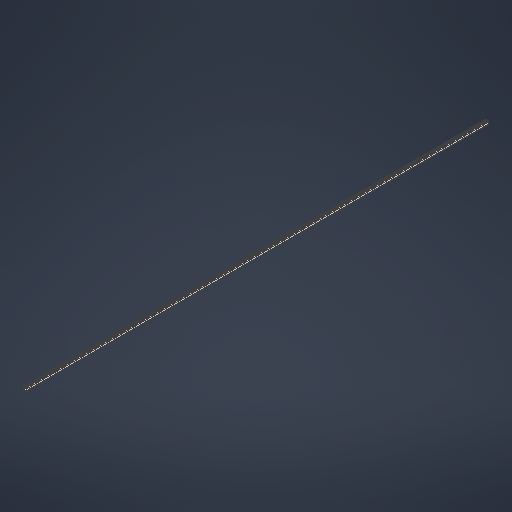
# Autodesk Inventor part: SP40-02 HOJA PUERTA BATIENTE INT - EXT
Saved by Autodesk Inventor 2025 (Build 290162000, 162)
## iProperties
Created: 2026-01-18
Part Number: SP40-02 HOJA PUERTA BATIENTE INT - EXT
Material: Aluminio
Document SubType Name: Modeling
Designer: ROLANDO
Density: 2.7 g/cm^3
Appearance: Satinado
Author: ROLANDO
Autodesk Inventor part; units mm, degrees
ref_plane "YZ Plane" through (0, 0, 0) normal (1, 0, 0) x (0, 1, 0)
ref_plane "XZ Plane" through (0, 0, 0) normal (0, 1, 0) x (-1, 0, 0)
ref_plane "XY Plane" through (0, 0, 0) normal (0, 0, 1) x (1, 0, 0)
sketch "Boceto1" plane through (0, 0, 0) normal (0, 0, 1) x (1, 0, 0)
  line L0 (33.1157, -5.4655) -> (33.1157, 13.4345)
  line L1 (32.6157, 13.9345) -> (-3.8843, 13.9345)
  line L2 (-4.3843, 13.4345) -> (-4.3843, -5.4655)
  line L3 (-3.8843, 15.3345) -> (32.6157, 15.3345)
  line L4 (34.5157, 29.7345) -> (34.5157, -11.2655)
  line L5 (-5.7843, -28.8655) -> (-5.7843, 25.5945)
  line L6 (33.1157, 15.8345) -> (33.1157, 28.3345)
  line L7 (34.5157, 29.7345) -> (20.3157, 29.7345)
  line L8 (20.3157, 29.7345) -> (20.3157, 28.0945)
  line L9 (24.1157, 28.3345) -> (24.1157, 21.8345)
  line L10 (25.5157, 20.4345) -> (25.5157, 28.3345)
  line L11 (25.5157, 20.4345) -> (20.3157, 20.4345)
  line L12 (20.3157, 20.4345) -> (20.3157, 22.0745)
  line L13 (21.7157, 21.8345) -> (24.1157, 21.8345)
  line L14 (21.7157, 23.0845) -> (21.0099, 23.0845)
  line L15 (21.0099, 23.0845) -> (20.3157, 22.0745)
  line L16 (21.7157, 27.0845) -> (21.0099, 27.0845)
  line L17 (-4.3843, 15.8345) -> (-4.3843, 22.8345)
  line L18 (-4.3843, 22.8345) -> (-2.8843, 22.8345)
  line L19 (-2.8843, 22.8345) -> (-2.8843, 25.5945)
  line L20 (-1.6443, 29.7345) -> (6.5157, 29.7345)
  line L21 (5.0777, 28.3345) -> (-0.1443, 28.3345)
  line L22 (6.5157, 29.7345) -> (6.5157, 27.2345)
  line L23 (6.5157, 27.2345) -> (5.8057, 27.2345)
  line L24 (5.8057, 27.2345) -> (5.0777, 28.3345)
  line L25 (33.1157, -7.8655) -> (33.1157, -11.2655)
  line L26 (33.6157, -11.7655) -> (34.0157, -11.7655)
  line L27 (22.5157, -7.3655) -> (22.5157, -10.3655)
  line L28 (23.9157, -11.7655) -> (23.9157, -7.8655)
  line L29 (1.1157, -7.8655) -> (1.1157, -11.7655)
  line L30 (2.5157, -10.3655) -> (2.5157, -7.3655)
  line L31 (2.5157, -10.3655) -> (5.0157, -10.3655)
  line L32 (5.0157, -10.3655) -> (5.0157, -11.7655)
  line L33 (5.0157, -11.7655) -> (1.1157, -11.7655)
  line L34 (22.5157, -10.3655) -> (20.0157, -10.3655)
  line L35 (20.0157, -10.3655) -> (20.0157, -11.7655)
  line L36 (20.0157, -11.7655) -> (23.9157, -11.7655)
  line L37 (21.4157, -5.4655) -> (21.4157, -4.5655)
  line L38 (21.4157, -4.5655) -> (3.6157, -4.5655)
  line L39 (-3.8843, -5.9655) -> (3.1157, -5.9655)
  line L40 (21.9157, -5.9655) -> (32.6157, -5.9655)
  line L41 (20.0157, -7.3655) -> (20.0157, -5.9655)
  line L42 (5.0157, -5.9655) -> (5.0157, -7.3655)
  line L43 (21.7157, 28.3345) -> (24.1157, 28.3345)
  line L44 (25.5157, 28.3345) -> (33.1157, 28.3345)
  line L45 (32.6157, -7.3655) -> (24.4157, -7.3655)
  line L46 (5.0157, -7.3655) -> (2.5157, -7.3655)
  line L47 (0.6157, -7.3655) -> (-4.3843, -7.3655)
  line L48 (22.5157, -7.3655) -> (20.0157, -7.3655)
  line L49 (22.5157, -7.3655) -> (20.0157, -7.3655)
  line L50 (3.6157, -4.5655) -> (3.6157, -5.4655)
  line L51 (5.0157, -5.9655) -> (20.0157, -5.9655)
  line L52 (20.3157, 28.0945) -> (21.0099, 27.0845)
  line L53 (21.7157, 28.3345) -> (21.7157, 27.0845)
  line L54 (21.7157, 21.8345) -> (21.7157, 23.0845)
  line L55 (-4.2843, -30.3655) -> (-3.3843, -30.3655)
  line L56 (-3.7843, -28.9655) -> (-3.8843, -28.9655)
  line L57 (-3.8843, -23.7655) -> (-3.7843, -23.7655)
  line L58 (-3.3843, -22.3655) -> (-4.3843, -22.3655)
  line L59 (-3.2843, -24.2655) -> (-3.2843, -24.3655)
  line L60 (-2.7843, -24.8655) -> (-2.3843, -24.8655)
  line L61 (-1.8843, -24.3655) -> (-1.8843, -23.8655)
  line L62 (-3.2843, -28.4655) -> (-3.2843, -28.3655)
  line L63 (-2.7843, -27.8655) -> (-2.3843, -27.8655)
  line L64 (-1.8843, -28.3655) -> (-1.8843, -28.8655)
  line L65 (-4.3843, -7.3655) -> (-4.3843, -22.3655)
  line L66 (-4.3843, -24.2655) -> (-4.3843, -28.4655)
  arc A0 (-1.8843, -23.8655) -> (-3.3843, -22.3655) centre (-3.3843, -23.8655) ccw
  arc A1 (-1.6443, 29.7345) -> (-5.7843, 25.5945) centre (-1.6443, 25.5945) ccw
  arc A2 (-0.1443, 28.3345) -> (-2.8843, 25.5945) centre (-0.1443, 25.5945) ccw
  arc A3 (-2.7843, -27.8655) -> (-3.2843, -28.3655) centre (-2.7843, -28.3655) ccw
  arc A4 (-1.8843, -28.3655) -> (-2.3843, -27.8655) centre (-2.3843, -28.3655) ccw
  arc A5 (-3.2843, -24.3655) -> (-2.7843, -24.8655) centre (-2.7843, -24.3655) ccw
  arc A6 (-2.3843, -24.8655) -> (-1.8843, -24.3655) centre (-2.3843, -24.3655) ccw
  arc A7 (1.1157, -7.8655) -> (0.6157, -7.3655) centre (0.6157, -7.8655) ccw
  arc A8 (3.1157, -5.9655) -> (3.6157, -5.4655) centre (3.1157, -5.4655) ccw
  arc A9 (-4.3843, -5.4655) -> (-3.8843, -5.9655) centre (-3.8843, -5.4655) ccw
  arc A10 (24.4157, -7.3655) -> (23.9157, -7.8655) centre (24.4157, -7.8655) ccw
  arc A11 (21.4157, -5.4655) -> (21.9157, -5.9655) centre (21.9157, -5.4655) ccw
  arc A12 (32.6157, -5.9655) -> (33.1157, -5.4655) centre (32.6157, -5.4655) ccw
  arc A13 (33.1157, -7.8655) -> (32.6157, -7.3655) centre (32.6157, -7.8655) ccw
  arc A14 (33.1157, -11.2655) -> (33.6157, -11.7655) centre (33.6157, -11.2655) ccw
  arc A15 (34.0157, -11.7655) -> (34.5157, -11.2655) centre (34.0157, -11.2655) ccw
  arc A16 (-4.3843, 15.8345) -> (-3.8843, 15.3345) centre (-3.8843, 15.8345) ccw
  arc A17 (-3.8843, 13.9345) -> (-4.3843, 13.4345) centre (-3.8843, 13.4345) ccw
  arc A18 (33.1157, 13.4345) -> (32.6157, 13.9345) centre (32.6157, 13.4345) ccw
  arc A19 (32.6157, 15.3345) -> (33.1157, 15.8345) centre (32.6157, 15.8345) ccw
  arc A20 (-3.2843, -24.2655) -> (-3.7843, -23.7655) centre (-3.7843, -24.2655) ccw
  arc A21 (-3.8843, -23.7655) -> (-4.3843, -24.2655) centre (-3.8843, -24.2655) ccw
  arc A22 (-4.3843, -28.4655) -> (-3.8843, -28.9655) centre (-3.8843, -28.4655) ccw
  arc A23 (-3.7843, -28.9655) -> (-3.2843, -28.4655) centre (-3.7843, -28.4655) ccw
  arc A24 (-5.7843, -28.8655) -> (-4.2843, -30.3655) centre (-4.2843, -28.8655) ccw
  arc A25 (-3.3843, -30.3655) -> (-1.8843, -28.8655) centre (-3.3843, -28.8655) ccw
  point P0 (-2.8843, 28.3345)
  point P1 (-5.7843, 29.7345)
  point P2 (22.9157, 20.4345)
  point P3 (-4.3843, -28.9655)
  point P4 (-4.3843, -23.7655)
  point P5 (-1.8843, -22.3655)
  point P6 (-3.2843, -23.7655)
  point P7 (-3.2843, -28.9655)
  point P8 (1.1157, -7.3655)
  point P9 (3.6157, -5.9655)
  point P10 (-4.3843, -5.9655)
  point P11 (23.9157, -7.3655)
  point P12 (21.4157, -5.9655)
  point P13 (33.1157, -5.9655)
  point P14 (33.1157, -7.3655)
  point P15 (-4.3843, 13.9345)
  point P16 (33.1157, 13.9345)
  point P17 (33.1157, 15.3345)
  point P18 (-4.3843, 15.3345)
  point P19 (3.6157, -5.0155)
  point P20 (-4.3843, -26.3655)
  point P21 (-1.8843, -30.3655)
  point P22 (-5.7843, -30.3655)
  point P23 (24.1157, 25.0845)
  dimension "d143" = 22.7
  dimension "d144" = 14.4
  dimension "d148" = 1.4
  dimension "d149" = 1.4
  dimension "d152" = 1.4
  dimension "d153" = 1.4
  dimension "d154" = 1.4
  dimension "d156" = 1.4
  dimension "d157" = 1.4
  dimension "d158" = 41.5
  dimension "d162" = 9.3
  dimension "d163" = 6.5
  dimension "d167" = 1.4
  dimension "d168" = 1.4
  dimension "d169" = 2.5
  dimension "d172" = 1.4
  dimension "d178" = 3
  dimension "d182" = 1.4
  dimension "d183" = 1.4
  dimension "d186" = 1.4
  dimension "d189" = 18.5
  dimension "d191" = 1.4
  dimension "d193" = 1.4
  dimension "d194" = 1.4
  dimension "d196" = 23
  dimension "d197" = 5.2
  dimension "d199" = 40.3
  dimension "d200" = 14.2
  dimension "d202" = 13.8
  dimension "d203" = 1.4
  dimension "d204" = 7.5
  dimension "d205" = 14.4
  dimension "d206" = 37.5
  dimension "d207" = 60.1
  dimension "d208" = 15
  dimension "d209" = 20
  dimension "d210" = 22.8
  dimension "d211" = 2.9
  dimension "d216" = 1.4
  dimension "d217" = 1.4
  dimension "d220" = 1.4
  dimension "d222" = 1.4
  dimension "d223" = 2.5
  dimension "d224" = 2.5
  dimension "d225" = 6.9
  dimension "d226" = 3
  dimension "d227" = 8
  dimension "d230" = 1.1
  dimension "d231" = 1.4
  dimension "d232" = 3
  dimension "d233" = 1.5
  dimension "d234" = 1.5
  dimension "d235" = 6.9
  dimension "d237" = 4.14
  dimension "d238" = 2.74
  dimension "d239" = 0.71
  dimension "d240" = 33.5
  dimension "d241" = 19.9
  dimension "d242" = 6.02
  dimension "d243" = 3.01
  dimension "d244" = 2.4
  dimension "d245" = 4
  dimension "d246" = 2
  dimension "d250" = 111
  constraints: 134 end point, 53 tangent, 52 point on circle, 43 point on line, 32 perpendicular, 26 centre point, 20 equal radius, 14 collinear, 7 vertical, 4 horizontal, 4 midpoint, 3 parallel
  measures "d143" distance between parallel lines of L45 L3
  measures "d144" distance between parallel lines of L3 L7
  measures "d148" distance between parallel lines of L7 L43
  measures "d149" distance between parallel lines of L7 L44
  measures "d152" distance between parallel lines of L4 L25
  measures "d153" distance between parallel lines of L10 L9
  measures "d154" distance between parallel lines of L11 L13
  measures "d156" distance between parallel lines of L12 L54
  measures "d157" distance between parallel lines of L8 L53
  measures "d158" distance between parallel lines of L26 L7
  measures "d162" distance between parallel lines of L7 L11
  measures "d163" distance between parallel lines of L13 L43
  measures "d167" distance between parallel lines of L17 L5
  measures "d168" distance between parallel lines of L20 L21
  measures "d169" distance of L20.end L22.end
  measures "d172" distance between parallel lines of L51 L38
  measures "d178" distance between parallel lines of L34 L48
  measures "d182" distance between parallel lines of L28 L27
  measures "d183" distance between parallel lines of L30 L29
  measures "d186" distance between parallel lines of L39 L47
  measures "d189" distance between parallel lines of L38 L1
  measures "d191" distance between parallel lines of L1 L3
  measures "d193" distance between parallel lines of L57 L58
  measures "d194" distance between parallel lines of L61 L59
  measures "d196" distance between parallel lines of L55 L47
  measures "d197" distance between parallel lines of L56 L57
  measures "d199" distance between parallel lines of L4 L5
  measures "d200" distance between parallel lines of L4 L8
  measures "d202" distance between parallel lines of L8 L22
  measures "d203" distance between parallel lines of L45 L40
  measures "d204" distance between parallel lines of L3 L18
  measures "d205" distance between parallel lines of L3 L20
  measures "d206" distance between parallel lines of L6 L17
  measures "d207" distance between parallel lines of L55 L20
  measures "d208" distance between parallel lines of L41 L42
  measures "d209" distance between parallel lines of L27 L30
  measures "d210" distance between parallel lines of L28 L29
  measures "d211" distance between parallel lines of L5 L19
  measures "d216" distance between parallel lines of L33 L31
  measures "d217" distance between parallel lines of L34 L36
  measures "d220" distance between parallel lines of L42 L50
  measures "d222" distance between parallel lines of L41 L37
  measures "d223" distance of L42.end L30.end
  measures "d224" distance of L27.start L41.start
  measures "d225" distance between parallel lines of L2 L30
  measures "d226" distance between parallel lines of L31 L46
  measures "d227" distance between parallel lines of L55 L58
  measures "d230" distance of point (-3.284, -28.966) point (-4.384, -28.966)
  measures "d231" distance between parallel lines of L55 L56
  measures "d232" distance between parallel lines of L63 L60
  measures "d233" distance from line of point (-4.384, -26.366) L60
  measures "d234" radius of A0
  measures "d235" distance between parallel lines of L18 L20
  measures "d237" radius of A1
  measures "d238" radius of A2
  measures "d239" distance of L22.end L23.end
  measures "d240" angle of L22 L24
  measures "d241" distance between parallel lines of L40 L1
  measures "d242" distance of L12.end L8.end
  measures "d243" vertical distance of L8.end point (24.116, 25.084)
  measures "d244" distance between parallel lines of L53 L9
  measures "d245" distance between parallel lines of L14 L16
  measures "d246" distance from line of point (24.116, 25.084) L16
  measures "d250" angle of L52 L15
extrude "Extrusión1" add sketch "Boceto1" against normal blind 5800
